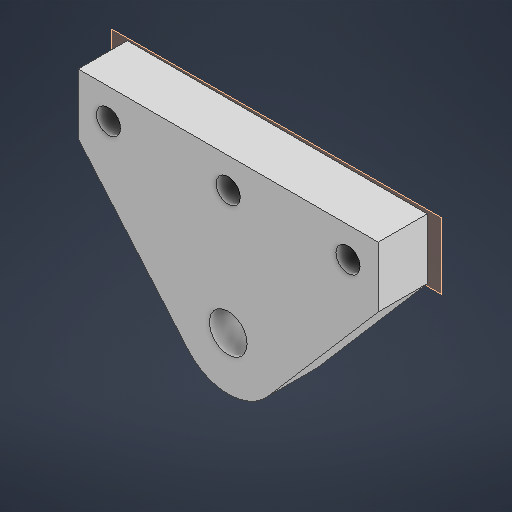
# Autodesk Inventor part: slider_02
Saved by Autodesk Inventor 2026 (Build 300175000, 175)
## iProperties
Created: 2025-12-05
Part Number: slider_02
Material: Generic
Document SubType Name: Modeling
Designer: numai
Density: 1 g/cm^3
Appearance: Default
Author: numai
Autodesk Inventor part; units mm, degrees
ref_plane "YZ Plane" through (0, 0, 0) normal (1, 0, 0) x (0, 1, 0)
ref_plane "XZ Plane" through (0, 0, 0) normal (0, 1, 0) x (-1, 0, 0)
ref_plane "XY Plane" through (0, 0, 0) normal (0, 0, 1) x (1, 0, 0)
ref_plane "作業平面1" through (-0.0753, -0.0002, 0) normal (0, 0, 1) x (0.9999894, 0.0046032, 0)
sketch "スケッチ1" plane through (-0.0753, -0.0002, 0) normal (0, 0, 1) x (0.9999894, 0.0046032, 0)
  line L0 (19.9118, -4.0915) -> (19.9486, 3.9084) projected
  line L1 (19.9486, 3.9084) -> (-19.7612, 4.0912) projected
  line L2 (-19.7612, 4.0912) -> (-19.7981, -3.9087) projected
  line L3 (-19.7981, -3.9087) -> (19.9118, -4.0915) projected
  circle A0 centre (-15.7797, 0.0728) radius 1.25 construction
  circle A1 centre (0.0753, -0.0002) radius 1.25 construction
  circle A2 centre (15.9302, -0.0732) radius 1.25 construction
  circle A3 centre (0, -16.35) radius 2.5 projected
  circle A4 centre (0, -16.35) radius 7
  line L4 (19.9118, -4.0915) -> (5.286, -20.9389)
  line L5 (-5.328, -20.8901) -> (-19.7981, -3.9087)
  circle A5 centre (15.9302, -0.0732) radius 1.6
  circle A6 centre (0.0753, -0.0002) radius 1.6
  circle A7 centre (-15.7797, 0.0728) radius 1.6
  point P0 (0.0753, -0.0002)
  dimension "d0" = 14
  dimension "d1" = 3.2
  constraints: 4 centre point, 4 coincident, 4 end point, 2 equal radius, 2 point on circle, 2 tangent
  measures "d0" diameter of A4
  measures "d1" diameter of A5
extrude "押し出し1" add sketch "スケッチ1" along normal blind 6.5
sketch "スケッチ2" plane through (-0.0753, -0.0002, 0) normal (0, 0, -1) x (-0.9999894, -0.0046032, 0)
  circle A0 centre (0, -16.35) radius 2.5 projected
  circle A1 centre (0, -16.35) radius 4
  point P0 (-0.0753, -0.0002)
  dimension "d4" = 8
  constraints: 1 centre point, 1 coincident
  measures "d4" diameter of A1
extrude "押し出し2" add sketch "スケッチ2" along normal blind 1
chamfer "面取り1" distance 1 angle 45 1 edges at (4, -16.3316, 0)
